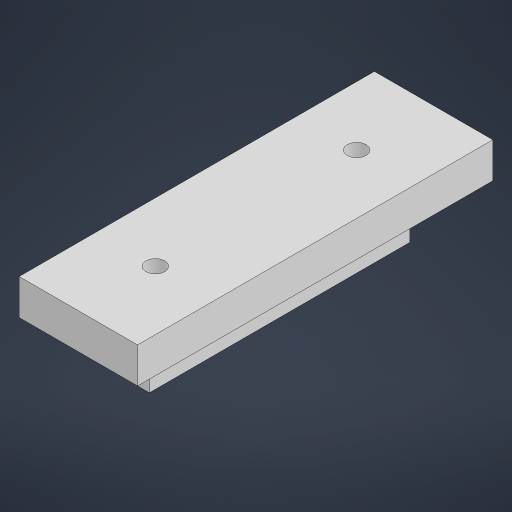
# Autodesk Inventor part: Zigu
Saved by Autodesk Inventor 2024.2 (Build 282272000, 272)
## iProperties
Created: 2024-03-05
Part Number: Zigu
Material: 一般
Document SubType Name: Modeling
Designer: Hanaoka
Density: 1 g/cm^3
Appearance: 既定
Author: Hanaoka
Autodesk Inventor part; units mm, degrees
ref_plane "YZ Plane" through (0, 0, 0) normal (1, 0, 0) x (0, 1, 0)
ref_plane "XZ Plane" through (0, 0, 0) normal (0, 1, 0) x (-1, 0, 0)
ref_plane "XY Plane" through (0, 0, 0) normal (0, 0, 1) x (1, 0, 0)
sketch "スケッチ1" plane through (0, 0, 0) normal (0, 1, 0) x (-1, 0, 0)
  line L0 (-2, 11) -> (2, 11)
  line L1 (2, 11) -> (2, -11)
  line L2 (2, -11) -> (-2, -11)
  line L3 (-2, -11) -> (-2, 11)
  line L4 (-2, 11) -> (2, -11) construction
  line L5 (2, 11) -> (-2, -11) construction
  circle A0 centre (0, 8.5) radius 0.8
  line L6 (0, -15.4) -> (0, 15.4) construction
  circle A1 centre (0, -8.5) radius 0.8
  line L7 (2.8, 0) -> (-2.8, 0) projected
  point P0 (0, 0)
  dimension "d0" = 4
  dimension "d1" = 2.5
  dimension "d2" = 1.6
  dimension "d3" = 22
  constraints: 12 end point, 2 centre point, 2 midpoint, 2 parallel, 2 point on line, 1 horizontal, 1 perpendicular, 1 other
  measures "d0" distance of L0.start L0.end
  measures "d1" distance from line of L0 A0.centre
  measures "d2" diameter of A0
  measures "d3" distance of L0.end L1.end
extrude "押し出し1" add sketch "スケッチ1" along normal blind 4
sketch "スケッチ2" plane through (0, 4, 0) normal (0, 1, 0) x (1, 0, 0)
  line L0 (5, -15) -> (-5, -15)
  line L1 (-5, -15) -> (-5, 15)
  line L2 (-5, 15) -> (5, 15)
  line L3 (5, 15) -> (5, -15)
  line L4 (5, -15) -> (-5, 15) construction
  line L5 (-5, -15) -> (5, 15) construction
  line L6 (2, -11) -> (2, 11) projected
  line L7 (2, 11) -> (-2, 11) projected
  line L8 (-2, 11) -> (-2, -11) projected
  line L9 (-2, -11) -> (2, -11) projected
  circle A0 centre (0, 8.5) radius 0.8 projected
  circle A1 centre (0, -8.5) radius 0.8 projected
  point P0 (0, 0)
  dimension "d6" = 30
  dimension "d7" = 10
  constraints: 12 end point, 2 midpoint, 2 parallel, 1 horizontal, 1 perpendicular
  measures "d6" distance of L0.end L1.end
  measures "d7" distance of L1.end L2.end
extrude "押し出し2" add sketch "スケッチ2" along normal blind 3 contours L0 L1 L2 L3 | L9 L8 L7 L6
